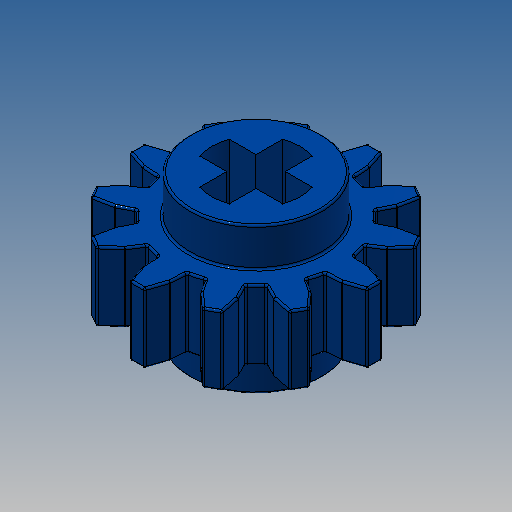
# Autodesk Inventor part: 69778-Blue
Saved by Autodesk Inventor 2025 (Build 290162010, 162A)
## iProperties
Created: 2014-08-13
Part Number: 69778-Blue
Material: ABS Plastic
Document SubType Name: Modeling
Designer: h.huther
Density: 1.06 g/cm^3
Appearance: Blau
Mass: 0.705537 g
Surface Area: 11.2279 cm^2
Volume: 0.665601 cm^3
Description: Technic, Gear 12
Author: h.muther
Autodesk Inventor part; units mm, degrees
ref_plane "YZ Plane" through (0, 0, 0) normal (1, 0, 0) x (0, 1, 0)
ref_plane "XZ Plane" through (0, 0, 0) normal (0, 1, 0) x (-1, 0, 0)
ref_plane "XY Plane" through (0, 0, 0) normal (0, 0, 1) x (1, 0, 0)
sketch "Sketch2" plane through (0, 0, 0) normal (0, 1, 0) x (-1, 0, 0)
  circle A0 centre (0, 0) radius 2.4 construction
  circle A1 centre (0, 0) radius 4.6336
  circle A2 centre (0, 0) radius 3.6
  circle A3 centre (0, 0) radius 3.6 construction
  line L0 (-0.8, 2.2627) -> (-0.8, 0.8)
  line L1 (-0.8, 0.8) -> (-2.2627, 0.8)
  line L2 (-2.2627, -0.8) -> (-0.8, -0.8)
  line L3 (-0.8, -0.8) -> (-0.8, -2.2627)
  line L4 (0.8, -2.2627) -> (0.8, -0.8)
  line L5 (0.8, -0.8) -> (2.2627, -0.8)
  line L6 (2.2627, 0.8) -> (0.8, 0.8)
  line L7 (0.8, 0.8) -> (0.8, 2.2627)
  arc A4 (0.8, 2.2627) -> (-0.8, 2.2627) centre (0, 0) ccw
  arc A5 (-2.2627, 0.8) -> (-2.2627, -0.8) centre (0, 0) ccw
  arc A6 (-0.8, -2.2627) -> (0.8, -2.2627) centre (0, 0) ccw
  arc A7 (2.2627, -0.8) -> (2.2627, 0.8) centre (0, 0) ccw
  line L8 (-3.6, 0.4) -> (-2.3664, 0.4)
  line L9 (-3.6, -0.4) -> (-2.3664, -0.4)
  arc A8 (-3.6, 0.4) -> (-3.6, -0.4) centre (-3.6, 0) ccw
  line L10 (2.3664, 0.4) -> (3.6, 0.4)
  arc A9 (3.6, -0.4) -> (3.6, 0.4) centre (3.6, 0) ccw
  line L11 (3.6, -0.4) -> (2.3664, -0.4)
  line L12 (-0.8, 4.564) -> (-0.75, 5.4496)
  line L13 (-0.75, 5.4496) -> (-0.4, 6.4976)
  line L14 (-0.4, 6.4976) -> (0.4, 6.4976)
  line L15 (0.4, 6.4976) -> (0.75, 5.4496)
  line L16 (0.75, 5.4496) -> (0.8, 4.564)
  point P0 (0, 6.4976)
  point P1 (-3.5777, -0.4)
  point P2 (-3.5777, 0.4)
  point P3 (3.5777, -0.4)
  point P4 (3.5777, 0.4)
  dimension "d1" = 4.8
  dimension "d2" = 1.6
  dimension "d3" = 0.8
  dimension "d4" = 7.2
  dimension "d9" = 7.2
  dimension "d11" = 0.8
  dimension "d12" = 1.5
  dimension "d13" = 1.6
  dimension "d14" = 1.048
  dimension "d29" = 6.4976
  dimension "d30" = 1.864
  constraints: 34 end point, 20 point on circle, 9 centre point, 9 equal length, 4 coincident, 4 horizontal alignment, 4 parallel, 4 perpendicular, 4 tangent, 3 horizontal, 1 equal radius, 1 midpoint, 1 vertical, 1 vertical alignment, 18 other
  measures "d2" distance between parallel lines of L0 L7
  measures "d3" distance between parallel lines of L8 L9
  measures "d4" diameter of A3
  measures "d9" diameter of A2
  measures "d11" distance of L13.end L14.end
  measures "d12" distance of L15.end L12.end
  measures "d13" distance of L16.end L12.start
  measures "d14" distance from line of L15.end L14
  measures "d29" distance from line of A1.centre L14
  measures "d30" distance edge to line of A1 L14
extrude "Extrusion1" add sketch "Sketch2" along normal mid plane 3.8 contours A1 | A2 L11 A7 L10 | A2 L10 A9 L11 | L10 A7 L6 L7 A4 L0 L1 A5 L8 A2 | A2 L9 A5 L2 L3 A6 L4 L5 A7 L11 | L8 A5 L9 A2 | A2 L9 A8 L8
extrude "Extrusion2" add sketch "Sketch2" along normal mid plane 8 contours A2 L11 A7 L10 | L10 A7 L6 L7 A4 L0 L1 A5 L8 A2 | A2 L9 A5 L2 L3 A6 L4 L5 A7 L11 | L8 A5 L9 A2
extrude "Extrusion3" add sketch "Sketch2" along normal mid plane 3.8 contours A1 L12 L13 L14 L15 L16
fillet "Fillet1" radius 0.1 6 edges at (0.75, 0, 5.4496) (0.8, 0, 4.564) (0.4, 0, 6.4976) (-0.4, 0, 6.4976) (-0.75, 0, 5.4496) (-0.8, 0, 4.564)
pattern_circular "Circular Pattern1" count 12 over 360 about axis through (0, 0, 0) along (0, 1, 0) of "Extrusion3", "Fillet1"
fillet "Fillet2" radius 0.1 196 edges at (-1.8501, 1.9, 4.7508) (-1.5809, 1.9, 4.3785) (-3.2765, 1.9, 3.2765) (-1.1993, 1.9, 4.4757) (-3.0014, 1.9, 3.5584) (-3.1893, 1.9, 3.9777) (-3.4789, 1.9, 4.8571) (-3.2488, 1.9, 5.6271) (-2.4669, 1.9, 5.4414) (1.1993, 1.9, 4.4757) (3.2765, 1.9, 3.2765) (4.4757, 1.9, 1.1993) (4.4757, 1.9, -1.1993) (3.2765, 1.9, -3.2765) (1.1993, 1.9, -4.4757) (-1.1993, 1.9, -4.4757) (-3.2765, 1.9, -3.2765) (-4.4757, 1.9, -1.1993) (-4.4757, 1.9, 1.1993) (-0.8201, 1.9, 4.5823) (-0.7732, 1.9, 5.0394) (-0.5843, 1.9, 5.9458) (0, 1.9, 6.4976) (0.5843, 1.9, 5.9458) (0.7732, 1.9, 5.0394) (0.8201, 1.9, 4.5823) (1.5809, 1.9, 4.3785) (1.8501, 1.9, 4.7508) (2.4669, 1.9, 5.4414) (3.2488, 1.9, 5.6271) (3.4789, 1.9, 4.8571) (3.1893, 1.9, 3.9777) (3.0014, 1.9, 3.5584) (3.5584, 1.9, 3.0014) (3.9777, 1.9, 3.1893) (4.8571, 1.9, 3.4789) (5.6271, 1.9, 3.2488) (5.4414, 1.9, 2.4669) (4.7508, 1.9, 1.8501) (4.3785, 1.9, 1.5809) (4.5823, 1.9, 0.8201) (5.0394, 1.9, 0.7732) (5.9458, 1.9, 0.5843) (6.4976, 1.9, 0) (5.9458, 1.9, -0.5843) (5.0394, 1.9, -0.7732) (4.5823, 1.9, -0.8201) (4.3785, 1.9, -1.5809) (4.7508, 1.9, -1.8501) (5.4414, 1.9, -2.4669) (5.6271, 1.9, -3.2488) (4.8571, 1.9, -3.4789) (3.9777, 1.9, -3.1893) (3.5584, 1.9, -3.0014) (3.0014, 1.9, -3.5584) (3.1893, 1.9, -3.9777) (3.4789, 1.9, -4.8571) (3.2488, 1.9, -5.6271) (2.4669, 1.9, -5.4414) (1.8501, 1.9, -4.7508) (1.5809, 1.9, -4.3785) (0.8201, 1.9, -4.5823) (0.7732, 1.9, -5.0394) (0.5843, 1.9, -5.9458) (0, 1.9, -6.4976) (-0.5843, 1.9, -5.9458) (-0.7732, 1.9, -5.0394) (-0.8201, 1.9, -4.5823) (-5.4414, 1.9, 2.4669) (-5.6271, 1.9, 3.2488) (-4.8571, 1.9, 3.4789) (-3.9777, 1.9, 3.1893) (-3.5584, 1.9, 3.0014) (-1.5809, 1.9, -4.3785) (-1.8501, 1.9, -4.7508) (-2.4669, 1.9, -5.4414) (-3.2488, 1.9, -5.6271) (-3.4789, 1.9, -4.8571) (-3.1893, 1.9, -3.9777) (-3.0014, 1.9, -3.5584) (-3.5584, 1.9, -3.0014) (-3.9777, 1.9, -3.1893) (-4.8571, 1.9, -3.4789) (-5.6271, 1.9, -3.2488) (-5.4414, 1.9, -2.4669) (-4.7508, 1.9, -1.8501) (-4.3785, 1.9, -1.5809) (-4.5823, 1.9, -0.8201) (-5.0394, 1.9, -0.7732) (-5.9458, 1.9, -0.5843) (-6.4976, 1.9, 0) (-5.9458, 1.9, 0.5843) (-5.0394, 1.9, 0.7732) (-4.5823, 1.9, 0.8201) (-4.3785, 1.9, 1.5809) (-4.7508, 1.9, 1.8501) (-2.4669, -1.9, 5.4414) (-3.2488, -1.9, 5.6271) (-3.4789, -1.9, 4.8571) (-3.1893, -1.9, 3.9777) (-3.0014, -1.9, 3.5584) (-3.2765, -1.9, 3.2765) (-1.1993, -1.9, 4.4757) (-1.5809, -1.9, 4.3785) (-1.8501, -1.9, 4.7508) (-3.5584, -1.9, 3.0014) (-3.9777, -1.9, 3.1893) (-4.8571, -1.9, 3.4789) (-5.6271, -1.9, 3.2488) (-5.4414, -1.9, 2.4669) (-4.7508, -1.9, 1.8501) (-4.3785, -1.9, 1.5809) (-4.4757, -1.9, 1.1993) (-4.5823, -1.9, 0.8201) (-5.0394, -1.9, 0.7732) (-5.9458, -1.9, 0.5843) (-6.4976, -1.9, 0) (-5.9458, -1.9, -0.5843) (-5.0394, -1.9, -0.7732) (-4.5823, -1.9, -0.8201) (-4.4757, -1.9, -1.1993) (-4.3785, -1.9, -1.5809) (-4.7508, -1.9, -1.8501) (-5.4414, -1.9, -2.4669) (-5.6271, -1.9, -3.2488) (-4.8571, -1.9, -3.4789) (-3.9777, -1.9, -3.1893) (-3.5584, -1.9, -3.0014) (-3.2765, -1.9, -3.2765) (-3.0014, -1.9, -3.5584) (-3.1893, -1.9, -3.9777) (-3.4789, -1.9, -4.8571) (-3.2488, -1.9, -5.6271) (-2.4669, -1.9, -5.4414) (-1.8501, -1.9, -4.7508) (-1.5809, -1.9, -4.3785) (-1.1993, -1.9, -4.4757) (-0.8201, -1.9, -4.5823) (-0.7732, -1.9, -5.0394) (-0.5843, -1.9, -5.9458) (0, -1.9, -6.4976) (0.5843, -1.9, -5.9458) (0.7732, -1.9, -5.0394) (0.8201, -1.9, -4.5823) (1.1993, -1.9, -4.4757) (1.5809, -1.9, -4.3785) (1.8501, -1.9, -4.7508) (2.4669, -1.9, -5.4414) (3.2488, -1.9, -5.6271) (3.4789, -1.9, -4.8571) (3.1893, -1.9, -3.9777) (3.0014, -1.9, -3.5584) (3.2765, -1.9, -3.2765) (3.5584, -1.9, -3.0014) (3.9777, -1.9, -3.1893) (4.8571, -1.9, -3.4789) (5.6271, -1.9, -3.2488) (-0.7732, -1.9, 5.0394) (-0.5843, -1.9, 5.9458) (0, -1.9, 6.4976) (0.5843, -1.9, 5.9458) (0.7732, -1.9, 5.0394) (0.8201, -1.9, 4.5823) (1.1993, -1.9, 4.4757) (1.5809, -1.9, 4.3785) (1.8501, -1.9, 4.7508) (2.4669, -1.9, 5.4414) (3.2488, -1.9, 5.6271) (3.4789, -1.9, 4.8571) (3.1893, -1.9, 3.9777) (3.0014, -1.9, 3.5584) (3.2765, -1.9, 3.2765) (3.5584, -1.9, 3.0014) (3.9777, -1.9, 3.1893) (4.8571, -1.9, 3.4789) (5.6271, -1.9, 3.2488) (5.4414, -1.9, 2.4669) (4.7508, -1.9, 1.8501) (4.3785, -1.9, 1.5809) (4.4757, -1.9, 1.1993) (4.5823, -1.9, 0.8201) (5.0394, -1.9, 0.7732) (5.9458, -1.9, 0.5843) (6.4976, -1.9, 0) (5.9458, -1.9, -0.5843) (5.0394, -1.9, -0.7732) (4.5823, -1.9, -0.8201) (4.4757, -1.9, -1.1993) (4.3785, -1.9, -1.5809) (4.7508, -1.9, -1.8501) (5.4414, -1.9, -2.4669) (-0.8201, -1.9, 4.5823) (3.5777, 1.9, 0.4) (3.5777, 4, 0.4) (3.5777, -4, 0.4) (3.5777, -1.9, 0.4)
equation "\"d1\" = kd"
equation "\"d2\" = axlet"
equation "\"d17\" = lu"
equation "\"kd\" = 4.8"
equation "\"axlet\" = 1.6"
equation "\"lu\" = 8"
body "Solid1"
